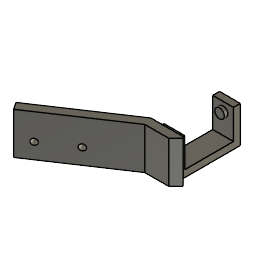
y chain mount (Autodesk Fusion 360 design; units mm, degrees)
Autodesk Fusion 360 part; units mm, degrees
note: some values were not read from the file. Set by a fixed rule: which sketch regions a step uses.
sketch "Szkic1" plane through (0, 0, 0) normal (0, 0, 1) x (1, 0, 0)
  line L0 (-44.8964, -16.5976) -> (-50, -20)
  line L1 (1.2574, 14.1716) -> (-43.5651, -15.7101)
  line L2 (10, 20) -> (2.5887, 15.0591)
  line L3 (25, 20) -> (10, 20)
  line L4 (35, 10) -> (25, 20)
  line L5 (35, -15) -> (35, 10)
  line L6 (35, -15) -> (-50, -15)
  line L7 (2.5887, 15.0591) -> (1.2574, 14.1716)
  constraint perpendicular L5 L6
  constraint parallel L1 L7
extrude "Wyciągnięcie proste1" add sketch "Szkic1" along normal blind 24.5
sketch "Szkic2" plane through (-6.1538, 9.2308, 0) normal (-0.5547, 0.83205, 0) x (-0.83205, -0.5547, 0)
  line L0 (-19.4145, 0) -> (43.6826, 0)
  line L1 (43.6826, 0) -> (43.6826, 24.5)
  line L2 (43.6826, 24.5) -> (-19.4145, 24.5)
  line L3 (-19.4145, 24.5) -> (-19.4145, 0)
extrude "Wyciągnięcie proste2" add 1 faces at (-2.0809, -5.2761, 24.5) along direction (0, 0, 1) blind 0.5
sketch "Szkic3" plane through (-6.1538, 9.2308, 0) normal (-0.5547, 0.83205, 0) x (-0.83205, -0.5547, 0)
  line L0 (-19.5, 9) -> (4.75, 9)
  line L1 (6.5, 10.75) -> (6.5, 25)
  line L2 (6.5, 9) -> (26.5, 9)
  circle A0 centre (26.5, 9) radius 1.75
  circle A1 centre (6.5, 9) radius 1.75
  line L3 (35, 0) -> (-19.45, 0)
  line L4 (-19.45, 0) -> (-19.45, 24)
  line L5 (-19.45, 24) -> (35, 24)
  line L6 (35, 24) -> (35, 0)
  dimension "d6" = 26
  dimension "d7" = 20
  dimension "d8" = 3.5
  dimension "d9" = 3.5
  constraint horizontal L0
  constraint perpendicular L0 L1
  constraint perpendicular L1 L2
  constraint coincident L2.end A0.centre
  constraint coincident L2.start A1.centre
  constraint coincident A1 L1.start
  constraint coincident A1 L0.end
  constraint perpendicular L3 L4
  constraint parallel L3 L5
  constraint parallel L4 L6
  constraint horizontal L3
  measures "d6" distance of L0.start L2.start
  measures "d7" distance of L2.start L2.end
  measures "d8" diameter of A0
  measures "d9" diameter of A1
extrude "Wyciągnięcie proste3" add sketch "Szkic3" along normal blind 5 contours L0 L1 A1 L4 L5 | L0 L1 A1 L3 L4 L5 L6
sketch "Szkic4" plane through (0, 20, 0) normal (0, 1, 0) x (-1, 0, 0)
  line L0 (-25, 0) -> (-10, 0)
  line L1 (-10, 0) -> (-10, 24)
  line L2 (-10, 24) -> (-10, 25)
  line L3 (-10, 25) -> (-25, 25)
  line L4 (-25, 25) -> (-25, 0)
  line L5 (-10, 0) -> (-25, 0)
  line L6 (-25, 0) -> (-25, 24)
  line L7 (-25, 24) -> (-10, 24)
  line L8 (-10, 24) -> (-10, 0)
  constraint perpendicular L5 L6
  constraint parallel L5 L7
  constraint parallel L6 L8
  constraint coincident L0.start L4.end
  constraint perpendicular L4 L5
  constraint coincident L0.end L1.start
extrude "Wyciągnięcie proste4" add sketch "Szkic4" along normal blind 5 contours L0 L1 L4 L5 L6 L7 L8
sketch "Szkic5" plane through (22.5, 22.5, 0) normal (0.707107, 0.707107, 0) x (-0.707107, 0.707107, 0)
  line L0 (-17.6777, 0) -> (-3.5355, 0)
  line L1 (-3.5355, 0) -> (-3.5355, 24)
  line L2 (-3.5355, 24) -> (-3.5355, 25)
  line L3 (-3.5355, 25) -> (-17.6777, 25)
  line L4 (-17.6777, 25) -> (-17.6777, 0)
  line L5 (-3.5355, 0) -> (-17.6777, 0)
  line L6 (-17.6777, 0) -> (-17.6777, 24)
  line L7 (-17.6777, 24) -> (-3.5355, 24)
  line L8 (-3.5355, 24) -> (-3.5355, 0)
  dimension "d14" = 24
  constraint perpendicular L5 L6
  constraint parallel L5 L7
  constraint parallel L6 L8
  constraint coincident L0.start L4.end
  constraint perpendicular L4 L5
  constraint coincident L0.end L1.start
  measures "d14" distance of L0.end L1.end
extrude "Wyciągnięcie proste5" add sketch "Szkic5" along normal blind 5 contours L0 L1 L4 L5 L6 L7 L8
extrude "Wyciągnięcie proste6" add 1 faces at (26.1785, 21.1785, 8) along direction (-0.707107, 0.707107, 0) blind 7
extrude "Wyciągnięcie proste7" add 1 faces at (9.0853, 21.436, 8) along direction (0.83205, 0.5547, 0) blind 8
extrude "Wyciągnięcie proste8" cut sketch "Szkic4" along normal blind 14 contours L0 L1 L4 L5 L6 L7 L8
extrude "Wyciągnięcie proste9" add sketch "Szkic4" along normal blind 5 contours L0 L1 L4 L5 L6 L7 L8
extrude "Wyciągnięcie proste10" cut 1 faces at (25, 26.3807, 8) along direction (1, 0, 0) blind 11
extrude "Wyciągnięcie proste11" cut 1 faces at (10, 25.3364, 8) along direction (-1, 0, 0) blind 5.5
extrude "Wyciągnięcie proste12" cut 1 faces at (0.8333, -3.3333, 25) along direction (0, 0, -1) blind 77
sketch "Szkic6" plane through (0, 25, 0) normal (0, 1, 0) x (-1, 0, 0)
  line L0 (-8.4861, 24) -> (-27.0711, 24)
  line L1 (-27.0711, 24) -> (-27.0711, 0)
  line L2 (-27.0711, 0) -> (-8.4861, 0)
  line L3 (-8.4861, 0) -> (-8.4861, 24)
  line L4 (-24, 21) -> (-12, 21)
  line L5 (-12, 21) -> (-12, 3)
  line L6 (-12, 3) -> (-24, 3)
  line L7 (-24, 3) -> (-24, 21)
  constraint perpendicular L4 L5
  constraint parallel L4 L6
  constraint parallel L5 L7
  constraint horizontal L4
extrude "Wyciągnięcie proste13" add sketch "Szkic6" along normal blind 36 contours L4 L5 L6 L7
sketch "Szkic7" plane through (0, 0, 21) normal (0, 0, 1) x (-1, 0, 0)
  line L0 (-12, -25) -> (-24, -25)
  line L1 (-24, -25) -> (-24, -61)
  line L2 (-24, -61) -> (-12, -61)
  line L3 (-12, -61) -> (-12, -25)
  line L4 (-24, -25) -> (-12, -25)
  line L5 (-12, -25) -> (-12, -29)
  line L6 (-12, -29) -> (-24, -29)
  line L7 (-24, -29) -> (-24, -25)
  line L8 (-24, -61) -> (-12, -61)
  line L9 (-12, -61) -> (-12, -57)
  line L10 (-12, -57) -> (-24, -57)
  line L11 (-24, -57) -> (-24, -61)
  dimension "d33" = 4
  dimension "d34" = 4
  constraint perpendicular L4 L5
  constraint parallel L4 L6
  constraint parallel L5 L7
  constraint coincident L0.start L3.end
  constraint perpendicular L3 L4
  constraint coincident L0.end L1.start
  constraint perpendicular L8 L9
  constraint parallel L8 L10
  constraint parallel L9 L11
  constraint coincident L2.end L3.start
  constraint perpendicular L3 L8
  constraint coincident L1.end L2.start
  measures "d33" distance of L0.end L6.end
  measures "d34" distance of L1.end L10.end
extrude "Wyciągnięcie proste14" cut sketch "Szkic7" against normal blind 17 contours L1 L3 L6 L10
extrude "Wyciągnięcie proste15" add 1 faces at (16, 37, 3) along direction (0, 0, -1) blind 3
sketch "Szkic8" plane through (0, 29, 0) normal (0, 1, 0) x (-1, 0, 0)
  line L0 (-12, 21) -> (-24, 21)
  line L1 (-24, 21) -> (-24, 4)
  line L2 (-24, 4) -> (-12, 4)
  line L3 (-12, 4) -> (-12, 21)
  circle A0 centre (-18, 16) radius 2.75
  dimension "d39" = 5.5
  measures "d39" diameter of A0
extrude "Wyciągnięcie proste16" add sketch "Szkic8" along normal blind 28 contours A0
extrude "Wyciągnięcie proste17" cut sketch "Szkic8" along normal blind 26 contours A0
extrude "Wyciągnięcie proste18" add sketch "Szkic8" along normal blind 2 contours A0
extrude "Wyciągnięcie proste19" cut 1 faces at (37.357, 12.357, 8) along direction (-0.707107, 0.707107, 0) blind 14
extrude "Wyciągnięcie proste20" cut 1 faces at (27.4575, 22.2565, 8) along direction (-0.707107, 0.707107, 0) blind 1
extrude "Wyciągnięcie proste21" cut 1 faces at (24.7978, 20.2022, 16) along direction (-0.707107, -0.707107, 0) blind 4.5
